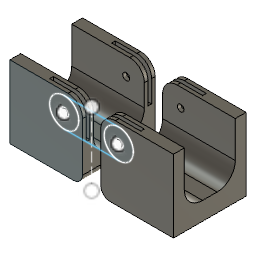
V0 - Multipart-box-test (Autodesk Fusion 360 design; units mm, degrees)
Autodesk Fusion 360 part; units mm, degrees
sketch "Sketch1" plane through (0, 0, 0) normal (0, 0, 1) x (1, 0, 0)
  line L0 (0, 0) -> (20, 0)
  line L1 (20, 0) -> (20, 20)
  line L2 (20, 20) -> (0, 20)
  line L3 (0, 20) -> (0, 0)
  line L4 (25, 0) -> (45, 0)
  line L5 (45, 0) -> (45, 20)
  line L6 (45, 20) -> (25, 20)
  line L7 (25, 20) -> (25, 0)
  dimension "d40" = 5
  constraint horizontal L0
  constraint vertical L1
  constraint horizontal L2
  constraint vertical L3
  constraint coincident L0.start L3.end
  constraint horizontal L4
  constraint vertical L5
  constraint horizontal L6
  constraint vertical L7
  measures "d40" distance of L1 L7
extrude "Extrude1" add sketch "Sketch1" along normal blind 20 makes body 1 at (0, 13.3333, 6.6667) makes body 2 at (25, 13.3333, 6.6667)
sketch "Sketch2" plane through (45, 0, 0) normal (1, 0, 0) x (0, 1, 0)
  line L0 (0, 0) -> (20, 0)
  line L1 (20, 0) -> (20, 20)
  line L2 (20, 20) -> (0, 20)
  line L3 (0, 20) -> (0, 0)
  line L4 (0, 20) -> (20, 20)
  line L5 (20, 20) -> (20, 0)
  line L6 (20, 0) -> (0, 0)
  line L7 (0, 0) -> (0, 20)
  line L8 (3, 20) -> (17, 20)
  line L9 (17, 20) -> (17, 10)
  line L10 (12, 5) -> (8, 5)
  line L11 (3, 10) -> (3, 20)
  arc A0 (3, 10) -> (8, 5) centre (8, 10) ccw
  arc A1 (12, 5) -> (17, 10) centre (12, 10) ccw
  dimension "d3" = 3
  dimension "d4" = 3
  dimension "d5" = 5
  dimension "d6" = 5
  constraint horizontal L4
  constraint vertical L5
  constraint horizontal L6
  constraint vertical L7
  constraint coincident L0.end L1.start
  constraint coincident L2.end L3.start
  constraint horizontal L8
  constraint vertical L9
  constraint horizontal L10
  constraint vertical L11
  constraint coincident L2 L8.start
  constraint tangent L11 A0
  constraint tangent L10 A0
  constraint tangent L9 A1
  constraint tangent L10 A1
  constraint equal A0 A1
  measures "d3" distance of L5 L9
  measures "d4" distance of L7 L11
  measures "d5" distance of L6 L10
  measures "d6" radius of A0
extrude "Extrude2" cut sketch "Sketch2" against normal blind 50 contours L2 L4 L8 L9 L10 L11 A0 A1 bodies 1 2
fillet "Fillet1" radius 2.5 2 edges at (20, 10, 0) (25, 10, 0) on bodies 1 2
sketch "Sketch3" plane through (0, 0, 0) normal (0, 1, 0) x (1, 0, 0)
  line L0 (0, -20) -> (50, -20)
  line L1 (50, -20) -> (50, 0)
  line L2 (50, 0) -> (0, 0)
  line L3 (0, 0) -> (0, -20)
  circle A0 centre (15, -15) radius 0.95
  circle A1 centre (30, -15) radius 0.9
  dimension "d11" = 1.9
  dimension "d12" = 1.8
  dimension "d41" = 15
  constraint horizontal L0
  constraint vertical L1
  constraint horizontal L2
  constraint vertical L3
  measures "d11" diameter of A0
  measures "d12" diameter of A1
  measures "d41" distance of A0.centre A1.centre
extrude "Extrude3" cut sketch "Sketch3" along normal up to surface (20 mm away) contours A0 | A1 bodies 1 2
sketch "Sketch4" plane through (0, 0, 20) normal (0, 0, 1) x (-1, 0, 0)
  line L0 (-20, -3) -> (0, -3)
  line L1 (0, -3) -> (0, 0)
  line L2 (0, 0) -> (-20, 0)
  line L3 (-20, 0) -> (-20, -3)
  line L4 (-35, -1) -> (-10, -1)
  line L5 (-10, -1) -> (-10, -2)
  line L6 (-10, -2) -> (-35, -2)
  line L7 (-35, -2) -> (-35, -1)
  line L8 (-35, -18) -> (-10, -18)
  line L9 (-10, -18) -> (-10, -19)
  line L10 (-10, -19) -> (-35, -19)
  line L11 (-35, -19) -> (-35, -18)
  point P0 (-25, 0)
  dimension "d15" = 10
  dimension "d16" = 10
  constraint horizontal L4
  constraint vertical L5
  constraint horizontal L6
  constraint vertical L7
  constraint horizontal L8
  constraint vertical L9
  constraint horizontal L10
  constraint vertical L11
  constraint collinear L5 L9
  constraint collinear L7 L11
  measures "d15" horizontal distance of L4.start P0
  measures "d16" distance of L3 L5
extrude "Extrude4" cut sketch "Sketch4" against normal blind 10 contours L3 L4 L6 L7 | L3 L4 L5 L6 | L8 L9 L10 L11 bodies 1 2
fillet "Fillet2" radius 4 8 edges at (20, 19.5, 20) (20, 17.5, 20) (20, 2.5, 20) (20, 0.5, 20) (25, 19.5, 20) (25, 17.5, 20) (25, 2.5, 20) (25, 0.5, 20) on bodies 1 2
fillet "Fillet3" radius 4 4 edges at (10, 1.5, 10) (10, 18.5, 10) (35, 18.5, 10) (35, 1.5, 10) on bodies 1 2
sketch "Sketch6" plane through (0, 0, 0) normal (0, -1, 0) x (1, 0, 0)
  arc A0 (20, 16) -> (16, 20) centre (16, 16) ccw
  line L0 (16, 20) -> (0, 20)
  line L1 (0, 20) -> (0, 0)
  line L2 (0, 0) -> (17.5, 0)
  arc A1 (17.5, 0) -> (20, 2.5) centre (17.5, 2.5) ccw
  line L3 (20, 2.5) -> (20, 16)
  circle A2 centre (15, 15) radius 0.95
  circle A3 centre (15, 15) radius 4
  circle A4 centre (15, 15) radius 1.15
  line L4 (22.5, 20) -> (22.5, 0) construction
  circle A5 centre (30, 15) radius 4
  circle A6 centre (30, 15) radius 1.15
  line L5 (15, 19) -> (30, 19)
  line L6 (15, 11) -> (30, 11)
  dimension "d23" = 8
  dimension "d24" = 0.2
  dimension "d42" = 15
  constraint concentric A2 A3
  constraint vertical L4
  constraint symmetric A3 L4 A5
  constraint symmetric A4 L4 A6
  constraint coincident A3 L5.start
  constraint coincident A5 L5.end
  constraint tangent A5 L5
  constraint coincident A3 L6.start
  constraint coincident A5 L6.end
  constraint tangent A5 L6
  measures "d23" diameter of A3
  measures "d42" distance of A2.centre A5.centre
extrude "Extrude5" [suppressed]
extrude "Extrude6" [suppressed]
fillet "Fillet6" [suppressed]
fillet "Fillet4" [suppressed]
fillet "Fillet5" [suppressed]
chamfer "Chamfer1" [suppressed]
chamfer "Chamfer2" [suppressed]
